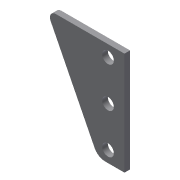
# Autodesk Inventor part: Belt plate mid
Saved by Autodesk Inventor 2015 SP1 (Build 190203100, 203)
## iProperties
Created: 2015-01-18
Part Number: Belt plate mid
Material: Generic
Document SubType Name: Sheet Metal
Designer: Owner
Density: 1 g/cm^3
Sheet Metal Rule: Default
Appearance: Default
Author: Owner
Autodesk Inventor part; units mm, degrees
ref_plane "YZ Plane" through (0, 0, 0) normal (1, 0, 0) x (0, 1, 0)
ref_plane "XZ Plane" through (0, 0, 0) normal (0, 1, 0) x (-1, 0, 0)
ref_plane "XY Plane" through (0, 0, 0) normal (0, 0, 1) x (1, 0, 0)
sketch "Sketch1" plane through (0, 0, 0) normal (0, 0, 1) x (1, 0, 0)
  line L0 (-50.8, 101.6) -> (101.6, 101.6)
  line L1 (50.8, 0) -> (101.6, 101.6)
  line L2 (-28, 56) -> (0, 0)
  line L3 (14.6239, 7) -> (34.6239, 7)
  line L4 (34.6239, 7) -> (34.6239, 2)
  line L5 (34.6239, 2) -> (14.6239, 2)
  line L6 (14.6239, 2) -> (14.6239, 7)
  line L7 (50.8, 0) -> (50.8, 62.4863)
  line L8 (14.6239, 14) -> (34.6239, 14)
  line L9 (34.6239, 14) -> (34.6239, 9)
  line L10 (34.6239, 9) -> (14.6239, 9)
  line L11 (14.6239, 9) -> (14.6239, 14)
  line L12 (14.6239, 21) -> (34.6239, 21)
  line L13 (34.6239, 21) -> (34.6239, 16)
  line L14 (34.6239, 16) -> (14.6239, 16)
  line L15 (14.6239, 16) -> (14.6239, 21)
  line L16 (14.6239, 28) -> (34.6239, 28)
  line L17 (34.6239, 28) -> (34.6239, 23)
  line L18 (34.6239, 23) -> (14.6239, 23)
  line L19 (14.6239, 23) -> (14.6239, 28)
  line L20 (14.6239, 35) -> (34.6239, 35)
  line L21 (34.6239, 35) -> (34.6239, 30)
  line L22 (34.6239, 30) -> (14.6239, 30)
  line L23 (14.6239, 30) -> (14.6239, 35)
  line L24 (14.6239, 42) -> (34.6239, 42)
  line L25 (34.6239, 42) -> (34.6239, 37)
  line L26 (34.6239, 37) -> (14.6239, 37)
  line L27 (14.6239, 37) -> (14.6239, 42)
  circle A0 centre (43.7057, 6.2222) radius 3.1623
  circle A1 centre (43.7057, 28) radius 3.1623
  circle A2 centre (43.7057, 49.7778) radius 3.1623
  line L28 (24.6239, 0) -> (24.6239, -15.6085)
  circle A3 centre (5.5421, 49.7778) radius 3.1623
  circle A4 centre (5.5421, 6.2222) radius 3.1623
  circle A5 centre (5.5421, 28) radius 3.1623
  line L29 (34.6239, 44) -> (14.6239, 44)
  line L30 (14.6239, 44) -> (14.6239, 49)
  line L31 (34.6239, 49) -> (34.6239, 44)
  line L32 (14.6239, 49) -> (34.6239, 49)
  line L33 (34.6239, 51) -> (14.6239, 51)
  line L34 (14.6239, 51) -> (14.6239, 56)
  line L35 (14.6239, 56) -> (34.6239, 56)
  line L36 (34.6239, 56) -> (34.6239, 51)
  circle A6 centre (-34.29, 91.44) radius 3.1623
  circle A7 centre (85.09, 91.44) radius 3.1623
  line L37 (14.6239, 0) -> (-28, 0)
  line L38 (-28, 0) -> (-28, 56)
  line L39 (-28, 56) -> (14.6239, 56)
  line L40 (14.6239, 56) -> (14.6239, 0)
  line L41 (-28, 56) -> (0, 0)
  line L42 (-28, 56) -> (14.6239, 56)
  line L43 (14.6239, 56) -> (14.6239, 0)
  line L44 (14.6239, 0) -> (0, 0)
  line L45 (0, 0) -> (14.6239, 0)
  line L46 (34.6239, 0) -> (50.8, 0)
  dimension "d8" = 50.8
  dimension "d9" = 152.4
  dimension "d11" = 50.8
  dimension "d12" = 20
  dimension "d13" = 5
  dimension "d15" = 7
  dimension "d16" = 6.3246
  dimension "d17" = 6.3246
  dimension "d18" = 6.3246
  dimension "d19" = 14
  dimension "d21" = 6.2222
  dimension "d24" = 6.3246
  dimension "d25" = 6.3246
  dimension "d26" = 34.29
  dimension "d27" = 34.29
  dimension "d28" = 10.16
  dimension "d29" = 10.16
  dimension "d40" = 9.0818
  dimension "d41" = 9.0818
  dimension "d42" = 9.0818
  dimension "d43" = 9.0818
  dimension "d44" = 9.0818
  dimension "d45" = 9.0818
  dimension "d46" = 26.1761
  measures "d8" distance of L2.end L1.start
  measures "d9" distance of L0.start L0.end
  measures "d11" horizontal distance of L0.end L1.start
  measures "d12" distance of L4.end L5.end
  measures "d13" distance between parallel lines of L3 L5
  measures "d15" distance of L3.start L8.start
  measures "d16" diameter of A0
  measures "d17" diameter of A1
  measures "d18" diameter of A2
  measures "d19" distance of L22.end L29.end
  measures "d21" distance from line of L35 A2.centre
  measures "d24" diameter of A6
  measures "d25" diameter of A7
  measures "d26" horizontal distance of A7.centre L1.start
  measures "d27" horizontal distance of A6.centre L2.end
  measures "d28" vertical distance of A6.centre L0.start
  measures "d29" vertical distance of A7.centre L0.end
  measures "d40" distance from line of L31 A2.centre
  measures "d41" distance from line of L30 A3.centre
  measures "d42" distance from line of L17 A1.centre
  measures "d43" distance from line of L4 A0.centre
  measures "d44" distance from line of L6 A4.centre
  measures "d45" distance from line of L19 A5.centre
  measures "d46" distance from line of L28 L1.start
extrude "Plate1" add sketch "Sketch1" along normal blind 3.048 contours L39 L34 L40 L30 L27 L23 L19 L15 L11 L6 L37 L2
sketch "Sketch2" plane through (0, 0, 3.048) normal (0, 0, 1) x (1, 0, 0)
  line L0 (14.6239, 56) -> (14.6239, 0) projected
  line L1 (-28, 56) -> (14.6239, 56) projected
  line L2 (14.6239, 0) -> (14.4969, 0)
  line L3 (14.4969, 0) -> (14.4969, 56)
  line L4 (14.4969, 56) -> (14.6239, 56)
  line L5 (14.6239, 56) -> (14.6239, 0)
  dimension "d33" = 0.127
  constraints: 8 end point, 2 parallel, 1 horizontal, 1 perpendicular, 1 point on line
  measures "d33" distance between parallel lines of L3 L0
extrude "Cut1" cut sketch "Sketch2" against normal blind 3.048
fillet "Corner Round1" radius 6.35 1 edges at (0, 0, 1.524)
fillet "Corner Round1" radius 3.175 1 edges at (-28, 56, 1.524)
equation "\"d17\" = d16"
equation "\"d18\" = d17"
equation "\"d21\" = 0.111111 * d20"
equation "\"d27\" = d26"
equation "\"d29\" = d28"
equation "\"d41\" = d40"
equation "\"d42\" = d40"
equation "\"d43\" = d42"
equation "\"d34\" = Thickness"
equation "\"BendRadius\" = Thickness"
equation "\"BendReliefWidth\" = Thickness"
equation "\"BendReliefDepth\" = 0.5 * Thickness"
equation "\"CornerReliefSize\" = 4 * Thickness"
equation "\"MinimumRemnant\" = 2 * Thickness"
equation "\"TransitionRadius\" = BendRadius"
equation "\"JacobiRadiusSize\" = BendRadius"
equation "\"GapSize\" = Thickness"
equation "\"d22\" = d21"
equation "\"d23\" = 0.5 * d20"
equation "\"d32\" = BendRadius"
equation "\"d20\" = 56"
equation "\"Thickness\" = 3.048"
body "Solid1"
